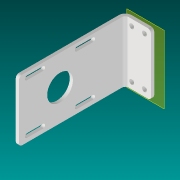
# Autodesk Inventor part: steppermount
Saved by Autodesk Inventor 2020.3 (Build 243373000, 373)
## iProperties
Created: 2020-05-24
Part Number: steppermount
Material: Aluminum 6061
Document SubType Name: Sheet Metal
Designer: Svend
Mass: 5.66404 g
Surface Area: 65.4079 cm^2
Volume: 5.66404 cm^3
Density: 2.7 g/cm^3
Sheet Metal Rule: Default_mm
Appearance: Aluminum - Polished
Author: Svend
Autodesk Inventor part; units mm, degrees
ref_plane "YZ Plane" through (0, 0, 0) normal (1, 0, 0) x (0, 1, 0)
ref_plane "XZ Plane" through (0, 0, 0) normal (0, 1, 0) x (-1, 0, 0)
ref_plane "XY Plane" through (0, 0, 0) normal (0, 0, 1) x (1, 0, 0)
ref_plane "Work Plane1" through (0, 0, 0) normal (0, 0, 1) x (1, 0, 0)
ref_plane "Work Plane2" through (0, 0, 0) normal (0, 0, 1) x (1, 0, 0)
sketch "Sketch4" plane through (0, 0, 0) normal (0, 0, 1) x (1, 0, 0)
  circle A0 centre (-8, -36) radius 1.5
  circle A1 centre (-8, -6) radius 1.5
  circle A2 centre (-15.9281, -36) radius 1.5
  circle A3 centre (-15.9281, -6) radius 1.5
  line L0 (-19.9281, -2) -> (1.2168, -2)
  line L1 (-19.9281, -40) -> (-19.9281, -2)
  line L2 (-0.2416, -40) -> (-19.9281, -40)
  line L3 (-0.2416, -40) -> (-0.2416, -30)
  line L4 (-0.2416, -30) -> (0, -30)
  line L5 (0, -5) -> (0, -30)
  spline S0 degree 3 poles (1.2168, -2) (1.1498, -2.0729) (1.0846, -2.1482) (0.788, -2.5121) (0.5885, -2.8262) (0.3051, -3.4054) (0.1887, -3.7185) (0.036, -4.3634) (0, -4.6952) (0, -5) knots 0 0 0 0 0.087816 0.087816 0.414412 0.414412 0.707206 0.707206 1 1 1 1
  line L6 (-19.9281, -2) -> (-3.9281, -2)
  line L7 (-3.9281, -2) -> (-3.9281, -40)
  line L8 (-3.9281, -40) -> (-19.9281, -40)
  line L9 (-19.9281, -40) -> (-19.9281, -2)
  point P0 (0, 0)
  dimension "d20" = 16
  measures "d20" distance between parallel lines of L9 L7
extrude "Plate3" add sketch "Sketch4" along normal blind 2 contours L0 L7 L2 L1
sketch "Sketch5" plane through (-19.9281, -40, 2) normal (-1, 0, 0) x (0, -1, 0)
  line L0 (-38, 0) -> (0, 0)
  line L1 (0, 0) -> (0, 66)
  line L2 (0, 66) -> (-38, 66)
  line L3 (-38, 66) -> (-38, 0)
  constraints: 6 end point, 1 horizontal, 1 perpendicular, 1 vertical
edge flange "Flange2" height 68 angle 90 thickness 2 bend radius 2 thickness toward (-1, 0, 0) relief straight relief width 2 relief depth 1 edges at (-19.9281, -21, 2) wall of the first edge with corners at (-19.9281, -2, 2) (-19.9281, -40, 2) (-19.9281, -40, 68) (-19.9281, -2, 68)
bend "Bend2"
corner "Corner2"
sketch "Sketch6" plane through (-21.9281, -40, 68) normal (-1, 0, 0) x (0, 0, 1)
  circle A0 centre (-41.0214, 34.5) radius 1.25 projected
  circle A1 centre (-41.0214, 3.5) radius 1.25 projected
  circle A2 centre (-10.0214, 34.5) radius 1.25 projected
  circle A3 centre (-10.0214, 3.5) radius 1.25 projected
  line L0 (-46.0214, 3.5) -> (-36.0214, 3.5) construction
  line L1 (-46.0214, 2) -> (-36.0214, 2)
  line L2 (-36.0214, 5) -> (-46.0214, 5)
  arc A4 (-46.0214, 5) -> (-46.0214, 2) centre (-46.0214, 3.5) ccw
  arc A5 (-36.0214, 2) -> (-36.0214, 5) centre (-36.0214, 3.5) ccw
  circle A6 centre (-25.5214, 19) radius 2.65 projected
  circle A7 centre (-25.5214, 19) radius 8
  line L3 (-46.0214, 34.5) -> (-36.0214, 34.5) construction
  line L4 (-46.0214, 33) -> (-36.0214, 33)
  line L5 (-36.0214, 36) -> (-46.0214, 36)
  arc A8 (-46.0214, 36) -> (-46.0214, 33) centre (-46.0214, 34.5) ccw
  arc A9 (-36.0214, 33) -> (-36.0214, 36) centre (-36.0214, 34.5) ccw
  line L6 (-15.0214, 34.5) -> (-5.0214, 34.5) construction
  line L7 (-15.0214, 33) -> (-5.0214, 33)
  line L8 (-5.0214, 36) -> (-15.0214, 36)
  arc A10 (-15.0214, 36) -> (-15.0214, 33) centre (-15.0214, 34.5) ccw
  arc A11 (-5.0214, 33) -> (-5.0214, 36) centre (-5.0214, 34.5) ccw
  line L9 (-15.0214, 3.5) -> (-5.0214, 3.5) construction
  line L10 (-15.0214, 2) -> (-5.0214, 2)
  line L11 (-5.0214, 5) -> (-15.0214, 5)
  arc A12 (-15.0214, 5) -> (-15.0214, 2) centre (-15.0214, 3.5) ccw
  arc A13 (-5.0214, 2) -> (-5.0214, 5) centre (-5.0214, 3.5) ccw
  line L12 (-30.5214, 19) -> (-20.5214, 19) construction
  line L13 (-30.5214, 27) -> (-20.5214, 27)
  line L14 (-20.5214, 11) -> (-30.5214, 11)
  arc A14 (-30.5214, 27) -> (-30.5214, 11) centre (-30.5214, 19) ccw
  arc A15 (-20.5214, 11) -> (-20.5214, 27) centre (-20.5214, 19) ccw
  point P0 (-68, 40)
  dimension "d32" = 5
  dimension "d33" = 16
  dimension "d34" = 5
  dimension "d37" = 5
  dimension "d39" = 3
  dimension "d40" = 3
  dimension "d41" = 3
  dimension "d42" = 3
  constraints: 40 end point, 21 tangent, 20 point on circle, 11 centre point, 8 parallel, 5 midpoint, 3 horizontal, 1 coincident, 1 point on line
  measures "d32" distance of A1.centre L0.end
  measures "d33" diameter of A7
  measures "d34" distance of A2.centre L6.end
  measures "d37" distance of A7.centre L12.end
  measures "d39" distance between parallel lines of L1 L2
  measures "d40" distance between parallel lines of L10 L11
  measures "d41" distance between parallel lines of L8 L7
  measures "d42" distance between parallel lines of L4 L5
extrude "Cut2" cut sketch "Sketch6" against normal blind 2 contours A0 | A1 | A2 | A3 | A4 L2 A5 L1 | A6 | A7 | A7 L13 A15 L14 | A7 L14 A14 L13 | A8 L5 A9 L4 | A10 L8 A11 L7 | A12 L11 A13 L10
fillet "Corner Round2" radius 2 4 edges at (-20.9281, -40, 68) (-20.9281, -2, 68) (-3.9281, -2, 1) (-3.9281, -40, 1)
equation "\"d40\" = d39"
equation "\"d41\" = d39"
equation "\"d42\" = d39"
equation "\"d35\" = Thickness"
equation "\"d21\" = Thickness"
equation "\"d22\" = BendReliefWidth"
equation "\"d23\" = BendReliefDepth"
equation "\"d24\" = MinimumRemnant"
equation "\"d25\" = TransitionRadius"
equation "\"d28\" = BendRadius"
equation "\"d29\" = CornerReliefSize"
equation "\"d30\" = GapSize"
equation "\"d31\" = JacobiRadiusSize"
equation "\"BendRadius\" = Thickness"
equation "\"BendReliefWidth\" = Thickness"
equation "\"BendReliefDepth\" = 0.5 * Thickness"
equation "\"CornerReliefSize\" = 4 * Thickness"
equation "\"MinimumRemnant\" = 2 * Thickness"
equation "\"TransitionRadius\" = BendRadius"
equation "\"JacobiRadiusSize\" = BendRadius"
equation "\"GapSize\" = Thickness"
equation "\"Thickness\" = 2"
body "Solid2"
